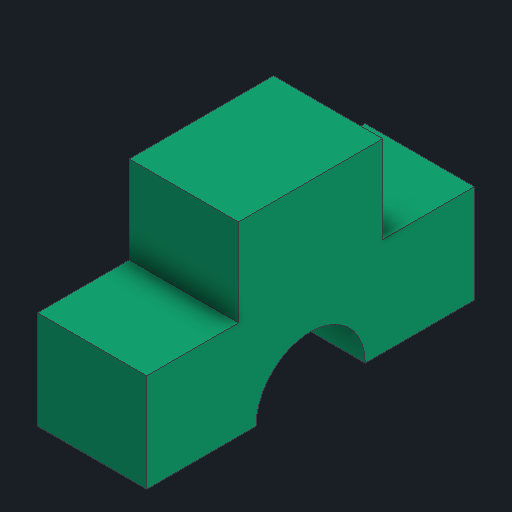
# Autodesk Inventor part: 110033226_ipt_18_大橋圍牆
Saved by Autodesk Inventor 2022 (Build 260153000, 153)
## iProperties
Created: 2022-06-23
Part Number: 110033226_ipt_18_大橋圍牆
Material: 一般
Document SubType Name: Modeling
Designer: User
Density: 1 g/cm^3
Appearance: 熔接 - 鋁
Author: User
Autodesk Inventor part; units mm, degrees
ref_plane "YZ Plane" through (0, 0, 0) normal (1, 0, 0) x (0, 1, 0)
ref_plane "XZ Plane" through (0, 0, 0) normal (0, 1, 0) x (-1, 0, 0)
ref_plane "XY Plane" through (0, 0, 0) normal (0, 0, 1) x (1, 0, 0)
sketch "草圖1" plane through (0, 0, 0) normal (0, 1, 0) x (-1, 0, 0)
  line L0 (2.5, 7.5) -> (-2.5, 7.5)
  line L1 (-2.5, 7.5) -> (-2.5, -7.5)
  line L2 (-2.5, -7.5) -> (2.5, -7.5)
  line L3 (2.5, -7.5) -> (2.5, 7.5)
  circle A0 centre (0, 0) radius 1.7
  circle A1 centre (0, 5) radius 1.7
  circle A2 centre (0, -5) radius 1.7
  point P0 (2.5, 0)
  point P1 (0, -7.5)
  dimension "d0" = 5
  dimension "d1" = 15
  dimension "d2" = 3.4
  dimension "d3" = 3.4
  dimension "d4" = 3.4
  dimension "d5" = 2.5
  dimension "d6" = 2.5
  constraints: 8 end point, 3 centre point, 3 vertical alignment, 2 midpoint, 2 parallel, 1 coincident, 1 horizontal, 1 horizontal alignment, 1 perpendicular
  measures "d0" distance of L2.end L1.end
  measures "d1" distance of L1.end L0.end
  measures "d2" diameter of A0
  measures "d3" diameter of A1
  measures "d4" diameter of A2
  measures "d5" distance from line of L2 A2.centre
  measures "d6" distance from line of L0 A1.centre
sketch "草圖2" plane through (0, 0, 0) normal (1, 0, 0) x (0, 1, 0)
  line L0 (0, 7.5) -> (0, -7.5) projected
  line L1 (0, 3.3) -> (0, 6.7) projected
  line L2 (0, -6.7) -> (0, -3.3) projected
  line L3 (0, -1.7) -> (0, 1.7) projected
  line L4 (0, 7.5) -> (4.5, 7.5)
  line L5 (4.5, 7.5) -> (4.5, -7.5)
  line L6 (4.5, -7.5) -> (0, -7.5)
  line L7 (4.5, 3.3) -> (8.5, 3.3)
  line L8 (8.5, 3.3) -> (8.5, -3.3)
  line L9 (8.5, -3.3) -> (4.5, -3.3)
  circle A0 centre (0, 0) radius 2.5
  point P0 (8.5, 0)
  point P1 (4.5, 0)
  point P2 (0, 2.5)
  point P3 (0, -2.5)
  dimension "d7" = 4.5
  dimension "d8" = 4
  dimension "d9" = 6.6
  dimension "d12" = 5
  constraints: 12 end point, 4 perpendicular, 2 horizontal, 2 midpoint, 2 point on line, 1 centre point, 1 coincident, 1 horizontal alignment, 1 other
  measures "d7" distance of L4.start L4.end
  measures "d8" distance of L7.start L7.end
  measures "d9" distance of L7.end L8.end
  measures "d12" diameter of A0
extrude "擠出1" add sketch "草圖2" along normal mid plane 5 contours L4 L5 L6 L0 A0 | L7 L8 L9 L5
extrude "擠出2" cut sketch "草圖1" along normal blind 1.5 contours A1 | A2
